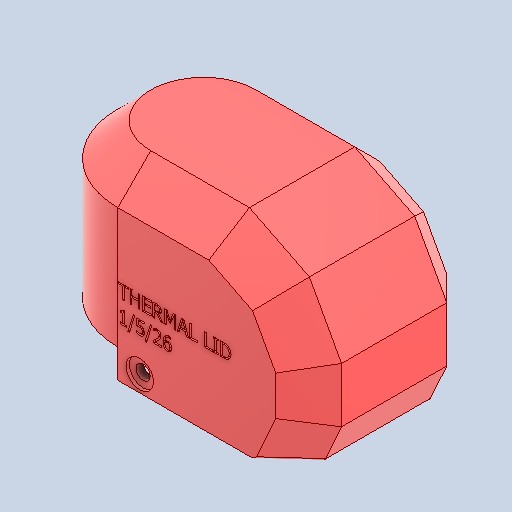
# Autodesk Inventor part: Thermal Lid
Saved by Autodesk Inventor 2026.2 (Build 302298000, 298)
## iProperties
Created: 2025-12-29
Part Number: Thermal Lid
Material: ABS Plastic
Document SubType Name: Modeling
Designer: mumin
Density: 1.06 g/cm^3
Appearance: Smooth - White
Author: mumin
Autodesk Inventor part; units mm, degrees
note: some values were not read from the file. Chosen so that the rebuilt part matches the saved one: direction of "Hole2".
ref_plane "YZ Plane" through (0, 0, 0) normal (1, 0, 0) x (0, 1, 0)
ref_plane "XZ Plane" through (0, 0, 0) normal (0, 1, 0) x (-1, 0, 0)
ref_plane "XY Plane" through (0, 0, 0) normal (0, 0, 1) x (1, 0, 0)
sketch "Sketch1" plane through (0, 0, 0) normal (0, 0, 1) x (1, 0, 0)
  line L0 (0, 0) -> (0, 70)
  line L1 (0, 70) -> (84, 70)
  line L2 (-25.2, 0) -> (151.2, 0) projected
  line L3 (0, 0) -> (100, 0)
  line L4 (126, 4.4656) -> (118.0459, -13.2)
  line L5 (84, 70) -> (111.3558, 56.3184)
  line L6 (111.3558, 56.3184) -> (126, 29.4656)
  line L7 (126, 29.4656) -> (126, 4.4656)
  line L8 (39, 0) -> (39, -13.2)
  line L9 (39, -13.2) -> (118.0459, -13.2)
  point P0 (123.9893, 0)
  dimension "d0" = 70
  dimension "d1" = 84
  dimension "d2" = 42
  dimension "d36" = 100
  dimension "d37" = 65.76
  dimension "d41" = 13.2
  dimension "d42" = 39
  constraints: 18 end point, 3 perpendicular, 2 vertical, 1 collinear, 1 equal length, 1 point on line
  measures "d0" distance of L0.start L0.end
  measures "d1" distance of L0.end L1.end
  measures "d2" horizontal distance of L1.end L4.start
  measures "d36" distance from line of L0 L3.end
  measures "d37" angle of L4 L2
  measures "d41" distance of L8.start L8.end
  measures "d42" distance from line of L8 L0.start
extrude "Bilateral Extrude" add sketch "Sketch1" along normal mid plane 78
sketch "Sketch2" plane through (0, 70, -39) normal (0, 1, 0) x (1, 0, 0)
  line L0 (0, -39) -> (126, -39)
  line L1 (126, 0) -> (126, -78) projected
  line L2 (84, -78) -> (0, -78) projected
  arc A0 (39, 0) -> (39, -78) centre (39, -39) ccw
  line L3 (39, -39) -> (39, 0) construction
  line L4 (39, -39) -> (39, -78) construction
  line L5 (0, 0) -> (0, -78) projected
  line L6 (39, 0) -> (0, 0)
  line L7 (0, -78) -> (39, -78)
  dimension "d6" = 180
  constraints: 10 end point, 2 perpendicular, 2 point on circle, 2 point on line, 2 tangent, 1 centre point, 1 collinear, 1 midpoint
  measures "d6" angle of L3 L4
extrude "Rounded Front" cut sketch "Sketch2" against normal through all
shell "Shell1" thickness 5 removed faces 3 at (28.8362, 0, -8.1054) at (39, -8.8, 13) at (65.3486, -13.2, -13)
chamfer "Inside Chamfer" distance 12 angle 45 11 edges at (60.9097, 65, 34) (5, 65, 0) (60.9097, 65, -34) (95.2681, 58.7739, 34) (114.3584, 40.3694, 34) (121, 16.8651, 34) (95.2681, 58.7739, -34) (114.3584, 40.3694, -34) (121, 16.8651, -34) (116.7812, -3.8303, -34) (116.7812, -3.8303, 34)
chamfer "Outside Chamfer" distance 15 angle 45 11 edges at (61.5, 70, 39) (0, 70, 0) (61.5, 70, -39) (97.6779, 63.1592, 39) (118.6779, 42.892, 39) (126, 16.9656, 39) (122.023, -4.3672, 39) (97.6779, 63.1592, -39) (118.6779, 42.892, -39) (126, 16.9656, -39) (122.023, -4.3672, -39)
sketch "Sketch6" plane through (0, 0, 39) normal (0, 0, 1) x (1, 0, 0)
  line L0 (39.1286, 25.8223) -> (99.692, 25.8223) construction
  line L1 (99.692, 25.8223) -> (99.692, 6.0243) construction
  line L2 (99.692, 6.0243) -> (39.1286, 6.0243) construction
  line L3 (39.1286, 6.0243) -> (39.1286, 25.8223) construction
  line L4 (41.1702, 19.7223) -> (41.1702, 25.1006)
  line L5 (41.1702, 25.1006) -> (39.1237, 25.1006)
  line L6 (39.1237, 25.1006) -> (39.1237, 25.8223)
  line L7 (39.1237, 25.8223) -> (44.0274, 25.8223)
  line L8 (44.0274, 25.8223) -> (44.0274, 25.1006)
  line L9 (44.0274, 25.1006) -> (41.9809, 25.1006)
  line L10 (41.9809, 25.1006) -> (41.9809, 19.7223)
  line L11 (41.9809, 19.7223) -> (41.1702, 19.7223)
  line L12 (49.0745, 19.7223) -> (48.2638, 19.7223)
  line L13 (48.2638, 19.7223) -> (48.2638, 22.708)
  line L14 (48.2638, 22.708) -> (45.456, 22.708)
  line L15 (45.456, 22.708) -> (45.456, 19.7223)
  line L16 (45.456, 19.7223) -> (44.6453, 19.7223)
  line L17 (44.6453, 19.7223) -> (44.6453, 25.8223)
  line L18 (44.6453, 25.8223) -> (45.456, 25.8223)
  line L19 (45.456, 25.8223) -> (45.456, 23.4298)
  line L20 (45.456, 23.4298) -> (48.2638, 23.4298)
  line L21 (48.2638, 23.4298) -> (48.2638, 25.8223)
  line L22 (48.2638, 25.8223) -> (49.0745, 25.8223)
  line L23 (49.0745, 25.8223) -> (49.0745, 19.7223)
  line L24 (50.3103, 19.7223) -> (50.3103, 25.8223)
  line L25 (50.3103, 25.8223) -> (54.1265, 25.8223)
  line L26 (54.1265, 25.8223) -> (54.1265, 25.1006)
  line L27 (54.1265, 25.1006) -> (51.121, 25.1006)
  line L28 (51.121, 25.1006) -> (51.121, 23.4298)
  line L29 (51.121, 23.4298) -> (53.9238, 23.4298)
  line L30 (53.9238, 23.4298) -> (53.9238, 22.708)
  line L31 (53.9238, 22.708) -> (51.121, 22.708)
  line L32 (51.121, 22.708) -> (51.121, 20.444)
  line L33 (51.121, 20.444) -> (54.1265, 20.444)
  line L34 (54.1265, 20.444) -> (54.1265, 19.7223)
  line L35 (54.1265, 19.7223) -> (50.3103, 19.7223)
  line L36 (59.7371, 19.7223) -> (58.6842, 19.7223)
  line L37 (58.6842, 19.7223) -> (56.7563, 22.1495)
  line L38 (56.7563, 22.1495) -> (55.827, 22.1495)
  line L39 (55.827, 22.1495) -> (55.827, 19.7223)
  line L40 (55.827, 19.7223) -> (55.0163, 19.7223)
  line L41 (55.0163, 19.7223) -> (55.0163, 25.8223)
  line L42 (55.0163, 25.8223) -> (56.5882, 25.8223)
  spline S0 degree 2 poles (56.5882, 25.8223) (57.1122, 25.8223) (57.8191, 25.7086) (58.1404, 25.501) knots 0 0 0 1 2 2 2
  spline S1 degree 2 poles (58.1404, 25.501) (58.4617, 25.2934) (58.8325, 24.6458) (58.8325, 24.1663) knots 0 0 0 1 2 2 2
  spline S2 degree 2 poles (58.8325, 24.1663) (58.8325, 23.499) (58.1503, 22.5943) (57.567, 22.3768) knots 0 0 0 1 2 2 2
  line L43 (57.567, 22.3768) -> (59.7371, 19.7223)
  spline S3 degree 2 poles (57.9872, 24.102) (57.9872, 24.369) (57.7993, 24.7793) (57.6016, 24.9127) knots 0 0 0 1 2 2 2
  spline S4 degree 2 poles (57.6016, 24.9127) (57.4286, 25.0264) (56.9689, 25.1204) (56.6327, 25.1204) knots 0 0 0 1 2 2 2
  line L44 (56.6327, 25.1204) -> (55.827, 25.1204)
  line L45 (55.827, 25.1204) -> (55.827, 22.8267)
  line L46 (55.827, 22.8267) -> (56.5388, 22.8267)
  spline S5 degree 2 poles (56.5388, 22.8267) (56.8898, 22.8267) (57.4484, 22.9503) (57.6412, 23.143) knots 0 0 0 1 2 2 2
  spline S6 degree 2 poles (57.6412, 23.143) (57.8191, 23.3111) (57.9872, 23.7857) (57.9872, 24.102) knots 0 0 0 1 2 2 2
  line L47 (65.4515, 19.7223) -> (64.6408, 19.7223)
  line L48 (64.6408, 19.7223) -> (64.6408, 24.977)
  line L49 (64.6408, 24.977) -> (63.0491, 21.403)
  line L50 (63.0491, 21.403) -> (62.5548, 21.403)
  line L51 (62.5548, 21.403) -> (60.9779, 24.977)
  line L52 (60.9779, 24.977) -> (60.9779, 19.7223)
  line L53 (60.9779, 19.7223) -> (60.2215, 19.7223)
  line L54 (60.2215, 19.7223) -> (60.2215, 25.8223)
  line L55 (60.2215, 25.8223) -> (61.3288, 25.8223)
  line L56 (61.3288, 25.8223) -> (62.8514, 22.4263)
  line L57 (62.8514, 22.4263) -> (64.3245, 25.8223)
  line L58 (64.3245, 25.8223) -> (65.4515, 25.8223)
  line L59 (65.4515, 25.8223) -> (65.4515, 19.7223)
  line L60 (66.0299, 19.7223) -> (68.0863, 25.8223)
  line L61 (68.0863, 25.8223) -> (69.0848, 25.8223)
  line L62 (69.0848, 25.8223) -> (71.1412, 19.7223)
  line L63 (71.1412, 19.7223) -> (70.2861, 19.7223)
  line L64 (70.2861, 19.7223) -> (69.7324, 21.4277)
  line L65 (69.7324, 21.4277) -> (67.4041, 21.4277)
  line L66 (67.4041, 21.4277) -> (66.8505, 19.7223)
  line L67 (66.8505, 19.7223) -> (66.0299, 19.7223)
  line L68 (69.51, 22.1198) -> (68.5658, 24.9918)
  line L69 (68.5658, 24.9918) -> (67.6266, 22.1198)
  line L70 (67.6266, 22.1198) -> (69.51, 22.1198)
  line L71 (75.254, 19.7223) -> (71.7196, 19.7223)
  line L72 (71.7196, 19.7223) -> (71.7196, 25.8223)
  line L73 (71.7196, 25.8223) -> (72.5303, 25.8223)
  line L74 (72.5303, 25.8223) -> (72.5303, 20.444)
  line L75 (72.5303, 20.444) -> (75.254, 20.444)
  line L76 (75.254, 20.444) -> (75.254, 19.7223)
  line L77 (82.0461, 19.7223) -> (78.5117, 19.7223)
  line L78 (78.5117, 19.7223) -> (78.5117, 25.8223)
  line L79 (78.5117, 25.8223) -> (79.3224, 25.8223)
  line L80 (79.3224, 25.8223) -> (79.3224, 20.444)
  line L81 (79.3224, 20.444) -> (82.0461, 20.444)
  line L82 (82.0461, 20.444) -> (82.0461, 19.7223)
  line L83 (84.8094, 19.7223) -> (82.4465, 19.7223)
  line L84 (82.4465, 19.7223) -> (82.4465, 20.3452)
  line L85 (82.4465, 20.3452) -> (83.2226, 20.3452)
  line L86 (83.2226, 20.3452) -> (83.2226, 25.1995)
  line L87 (83.2226, 25.1995) -> (82.4465, 25.1995)
  line L88 (82.4465, 25.1995) -> (82.4465, 25.8223)
  line L89 (82.4465, 25.8223) -> (84.8094, 25.8223)
  line L90 (84.8094, 25.8223) -> (84.8094, 25.1995)
  line L91 (84.8094, 25.1995) -> (84.0333, 25.1995)
  line L92 (84.0333, 25.1995) -> (84.0333, 20.3452)
  line L93 (84.0333, 20.3452) -> (84.8094, 20.3452)
  line L94 (84.8094, 20.3452) -> (84.8094, 19.7223)
  spline S7 degree 2 poles (90.6227, 22.7674) (90.6227, 21.9319) (89.9455, 20.5874) (89.377, 20.2117) knots 0 0 0 1 2 2 2
  spline S8 degree 2 poles (89.377, 20.2117) (88.9123, 19.92) (87.9583, 19.7223) (87.2168, 19.7223) knots 0 0 0 1 2 2 2
  line L95 (87.2168, 19.7223) -> (85.8129, 19.7223)
  line L96 (85.8129, 19.7223) -> (85.8129, 25.8223)
  line L97 (85.8129, 25.8223) -> (87.2019, 25.8223)
  spline S9 degree 2 poles (87.2019, 25.8223) (88.0621, 25.8223) (89.0408, 25.5653) (89.3869, 25.3379) knots 0 0 0 1 2 2 2
  spline S10 degree 2 poles (89.3869, 25.3379) (89.9751, 24.9473) (90.6227, 23.6571) (90.6227, 22.7674) knots 0 0 0 1 2 2 2
  spline S11 degree 2 poles (89.7774, 22.7772) (89.7774, 23.4792) (89.3127, 24.4728) (88.853, 24.7546) knots 0 0 0 1 2 2 2
  spline S12 degree 2 poles (88.853, 24.7546) (88.5267, 24.9473) (87.7902, 25.1204) (87.2415, 25.1204) knots 0 0 0 1 2 2 2
  line L98 (87.2415, 25.1204) -> (86.6236, 25.1204)
  line L99 (86.6236, 25.1204) -> (86.6236, 20.4242)
  line L100 (86.6236, 20.4242) -> (87.2415, 20.4242)
  spline S13 degree 2 poles (87.2415, 20.4242) (87.7803, 20.4242) (88.5959, 20.5973) (88.9271, 20.8296) knots 0 0 0 1 2 2 2
  spline S14 degree 2 poles (88.9271, 20.8296) (89.3523, 21.1163) (89.7774, 22.0654) (89.7774, 22.7772) knots 0 0 0 1 2 2 2
  line L101 (43.0288, 9.6788) -> (40.053, 9.6788)
  line L102 (40.053, 9.6788) -> (40.053, 10.3017)
  line L103 (40.053, 10.3017) -> (41.1603, 10.3017)
  line L104 (41.1603, 10.3017) -> (41.1603, 14.3898)
  line L105 (41.1603, 14.3898) -> (40.053, 14.3898)
  line L106 (40.053, 14.3898) -> (40.053, 14.9483)
  spline S15 degree 2 poles (40.053, 14.9483) (40.6808, 14.9483) (41.274, 15.3043) (41.3135, 15.7986) knots 0 0 0 1 2 2 2
  line L107 (41.3135, 15.7986) -> (41.9463, 15.7986)
  line L108 (41.9463, 15.7986) -> (41.9463, 10.3017)
  line L109 (41.9463, 10.3017) -> (43.0288, 10.3017)
  line L110 (43.0288, 10.3017) -> (43.0288, 9.6788)
  line L111 (46.6869, 16.0507) -> (44.2993, 8.354)
  line L112 (44.2993, 8.354) -> (43.6072, 8.354)
  line L113 (43.6072, 8.354) -> (45.9849, 16.0507)
  line L114 (45.9849, 16.0507) -> (46.6869, 16.0507)
  spline S16 degree 2 poles (51.0567, 11.6166) (51.0567, 11.1766) (50.775, 10.4252) (50.5179, 10.1484) knots 0 0 0 1 2 2 2
  spline S17 degree 2 poles (50.5179, 10.1484) (50.2609, 9.8716) (49.4946, 9.5503) (49.0201, 9.5503) knots 0 0 0 1 2 2 2
  spline S18 degree 2 poles (49.0201, 9.5503) (48.5851, 9.5503) (47.7348, 9.7431) (47.4234, 9.8963) knots 0 0 0 1 2 2 2
  line L115 (47.4234, 9.8963) -> (47.4234, 10.7614)
  line L116 (47.4234, 10.7614) -> (47.4827, 10.7614)
  spline S19 degree 2 poles (47.4827, 10.7614) (47.5767, 10.6922) (47.9276, 10.5142) (48.1402, 10.4351) knots 0 0 0 1 2 2 2
  spline S20 degree 2 poles (48.1402, 10.4351) (48.3824, 10.3511) (48.7828, 10.2572) (49.0349, 10.2572) knots 0 0 0 1 2 2 2
  spline S21 degree 2 poles (49.0349, 10.2572) (49.2821, 10.2572) (49.7468, 10.4351) (49.9148, 10.6279) knots 0 0 0 1 2 2 2
  spline S22 degree 2 poles (49.9148, 10.6279) (50.0681, 10.8108) (50.2262, 11.2953) (50.2262, 11.6215) knots 0 0 0 1 2 2 2
  spline S23 degree 2 poles (50.2262, 11.6215) (50.2262, 11.9478) (50.0483, 12.363) (49.8802, 12.5014) knots 0 0 0 1 2 2 2
  spline S24 degree 2 poles (49.8802, 12.5014) (49.7072, 12.6547) (49.1931, 12.7832) (48.8817, 12.7832) knots 0 0 0 1 2 2 2
  spline S25 degree 2 poles (48.8817, 12.7832) (48.5455, 12.7832) (47.8782, 12.6794) (47.6755, 12.6349) knots 0 0 0 1 2 2 2
  line L117 (47.6755, 12.6349) -> (47.6755, 15.7788)
  line L118 (47.6755, 15.7788) -> (51.0221, 15.7788)
  line L119 (51.0221, 15.7788) -> (51.0221, 15.062)
  line L120 (51.0221, 15.062) -> (48.4615, 15.062)
  line L121 (48.4615, 15.062) -> (48.4615, 13.4357)
  spline S26 degree 2 poles (48.4615, 13.4357) (48.6098, 13.4555) (48.8965, 13.4703) (49.0151, 13.4703) knots 0 0 0 1 2 2 2
  spline S27 degree 2 poles (49.0151, 13.4703) (49.4848, 13.4703) (50.1323, 13.3171) (50.4289, 13.0897) knots 0 0 0 1 2 2 2
  spline S28 degree 2 poles (50.4289, 13.0897) (50.7305, 12.8623) (51.0567, 12.1702) (51.0567, 11.6166) knots 0 0 0 1 2 2 2
  line L122 (54.4725, 16.0507) -> (52.0849, 8.354)
  line L123 (52.0849, 8.354) -> (51.3929, 8.354)
  line L124 (51.3929, 8.354) -> (53.7706, 16.0507)
  line L125 (53.7706, 16.0507) -> (54.4725, 16.0507)
  line L126 (58.9066, 9.6788) -> (55.1448, 9.6788)
  line L127 (55.1448, 9.6788) -> (55.1448, 10.5439)
  spline S29 degree 2 poles (55.1448, 10.5439) (55.5502, 10.9245) (56.2719, 11.6314) (56.6179, 12.012) knots 0 0 0 1 2 2 2
  spline S30 degree 2 poles (56.6179, 12.012) (57.3149, 12.7782) (57.8241, 13.6977) (57.8241, 14.1871) knots 0 0 0 1 2 2 2
  spline S31 degree 2 poles (57.8241, 14.1871) (57.8241, 14.4441) (57.6659, 14.8297) (57.5225, 14.9533) knots 0 0 0 1 2 2 2
  spline S32 degree 2 poles (57.5225, 14.9533) (57.3792, 15.0769) (57.0035, 15.2005) (56.7761, 15.2005) knots 0 0 0 1 2 2 2
  spline S33 degree 2 poles (56.7761, 15.2005) (56.5586, 15.2005) (56.1137, 15.0917) (55.911, 15.0077) knots 0 0 0 1 2 2 2
  spline S34 degree 2 poles (55.911, 15.0077) (55.738, 14.9385) (55.4167, 14.7407) (55.3178, 14.6715) knots 0 0 0 1 2 2 2
  line L128 (55.3178, 14.6715) -> (55.2733, 14.6715)
  line L129 (55.2733, 14.6715) -> (55.2733, 15.5415)
  spline S35 degree 2 poles (55.2733, 15.5415) (55.5254, 15.6651) (56.4301, 15.9073) (56.8354, 15.9073) knots 0 0 0 1 2 2 2
  spline S36 degree 2 poles (56.8354, 15.9073) (57.6906, 15.9073) (58.6545, 15.0027) (58.6545, 14.2316) knots 0 0 0 1 2 2 2
  spline S37 degree 2 poles (58.6545, 14.2316) (58.6545, 13.8707) (58.4865, 13.2676) (58.3382, 13.0106) knots 0 0 0 1 2 2 2
  spline S38 degree 2 poles (58.3382, 13.0106) (58.1899, 12.7436) (57.7598, 12.2197) (57.5225, 11.9675) knots 0 0 0 1 2 2 2
  spline S39 degree 2 poles (57.5225, 11.9675) (57.1369, 11.5474) (56.1928, 10.6477) (55.911, 10.3857) knots 0 0 0 1 2 2 2
  line L130 (55.911, 10.3857) -> (58.9066, 10.3857)
  line L131 (58.9066, 10.3857) -> (58.9066, 9.6788)
  spline S40 degree 2 poles (63.578, 11.6561) (63.578, 11.1865) (63.2666, 10.3906) (63.0046, 10.1237) knots 0 0 0 1 2 2 2
  spline S41 degree 2 poles (63.0046, 10.1237) (62.7327, 9.8419) (62.0506, 9.5503) (61.6403, 9.5503) knots 0 0 0 1 2 2 2
  spline S42 degree 2 poles (61.6403, 9.5503) (61.23, 9.5503) (60.5527, 9.8271) (60.2957, 10.1039) knots 0 0 0 1 2 2 2
  spline S43 degree 2 poles (60.2957, 10.1039) (59.9793, 10.4351) (59.6234, 11.5474) (59.6234, 12.3581) knots 0 0 0 1 2 2 2
  spline S44 degree 2 poles (59.6234, 12.3581) (59.6234, 13.1539) (59.9497, 14.4342) (60.2908, 14.9088) knots 0 0 0 1 2 2 2
  spline S45 degree 2 poles (60.2908, 14.9088) (60.622, 15.3735) (61.6699, 15.8925) (62.357, 15.8925) knots 0 0 0 1 2 2 2
  spline S46 degree 2 poles (62.357, 15.8925) (62.5597, 15.8925) (62.9156, 15.853) (63.0491, 15.8085) knots 0 0 0 1 2 2 2
  line L132 (63.0491, 15.8085) -> (63.0491, 15.0225)
  line L133 (63.0491, 15.0225) -> (63.0145, 15.0225)
  spline S47 degree 2 poles (63.0145, 15.0225) (62.9008, 15.0818) (62.4856, 15.1856) (62.2483, 15.1856) knots 0 0 0 1 2 2 2
  spline S48 degree 2 poles (62.2483, 15.1856) (61.487, 15.1856) (60.5527, 14.1574) (60.4638, 13.149) knots 0 0 0 1 2 2 2
  spline S49 degree 2 poles (60.4638, 13.149) (60.7554, 13.3517) (61.3684, 13.5741) (61.7342, 13.5741) knots 0 0 0 1 2 2 2
  spline S50 degree 2 poles (61.7342, 13.5741) (62.0901, 13.5741) (62.624, 13.4308) (62.9156, 13.2133) knots 0 0 0 1 2 2 2
  spline S51 degree 2 poles (62.9156, 13.2133) (63.2518, 12.9611) (63.578, 12.1801) (63.578, 11.6561) knots 0 0 0 1 2 2 2
  spline S52 degree 2 poles (62.7476, 11.6215) (62.7476, 11.9972) (62.5498, 12.5064) (62.3323, 12.6843) knots 0 0 0 1 2 2 2
  spline S53 degree 2 poles (62.3323, 12.6843) (62.1692, 12.8128) (61.7638, 12.8969) (61.5513, 12.8969) knots 0 0 0 1 2 2 2
  spline S54 degree 2 poles (61.5513, 12.8969) (61.2646, 12.8969) (60.7258, 12.7239) (60.4638, 12.5607) knots 0 0 0 1 2 2 2
  spline S55 degree 2 poles (60.4638, 12.5607) (60.4588, 12.4718) (60.4489, 12.3037) (60.4489, 12.1752) knots 0 0 0 1 2 2 2
  spline S56 degree 2 poles (60.4489, 12.1752) (60.4489, 11.5424) (60.6961, 10.7663) (60.8839, 10.5637) knots 0 0 0 1 2 2 2
  spline S57 degree 2 poles (60.8839, 10.5637) (61.057, 10.3709) (61.4327, 10.2176) (61.6452, 10.2176) knots 0 0 0 1 2 2 2
  spline S58 degree 2 poles (61.6452, 10.2176) (62.1395, 10.2176) (62.7476, 10.9196) (62.7476, 11.6215) knots 0 0 0 1 2 2 2
  point P0 (0, 0)
  constraints: 2 other
emboss "LABEL" sketch "Sketch6" operation cut depth 1 direction (0, 0, -1)
fillet "Fillet2" radius 2 6 edges at (105.9823, -13.2, 28) (112.5625, -13.2, 0) (105.9823, -13.2, -28) (109.8207, -13.2, 31.5) (118.0459, -13.2, 0) (109.8207, -13.2, -31.5)
sketch "Sketch7" plane through (0, 0, 39) normal (0, 0, 1) x (1, 0, 0)
  line L0 (39, 0) -> (39, -13.2) projected
  point P0 (0, 0)
  point P1 (49, -5.7)
  dimension "d51" = 10
  dimension "d52" = 5.7
  measures "d51" distance from line of L0 point (49, -5.7)
  measures "d52" vertical distance of L0.start point (49, -5.7)
hole "Hole2" at (49, -5.7, 39) direction (0, 0, -1) diameter 6.5 end up to surface counterbore diameter 12.5 counterbore depth 1.5
mirror "Mirror Hole" about plane through (0, 0, 0) normal (0, 0, 1) of "Hole2"
body "Solid1"
